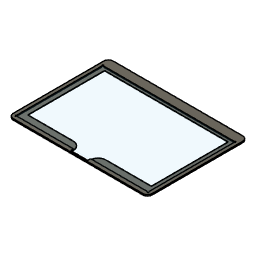
Pixsso_Assembly (Autodesk Fusion 360 archive; units mm, degrees)
design "PixssoFrame_ScreenBack"
Autodesk Fusion 360 part; units mm, degrees
sketch "Sketch1" plane through (0, 0, 0) normal (0, 0, 1) x (1, 0, 0)
  line L0 (90, 64.7) -> (-90, 64.7)
  line L1 (-90, 64.7) -> (-90, -64.7)
  line L2 (-90, -64.7) -> (90, -64.7)
  line L3 (90, -64.7) -> (90, 64.7)
  line L4 (90, 64.7) -> (-90, -64.7) construction
  line L5 (-90, 64.7) -> (90, -64.7) construction
  dimension "d1" = 129.4
  dimension "d2" = 180
  constraint horizontal L0
  constraint perpendicular L0 L1
  constraint parallel L0 L2
  constraint parallel L1 L3
  constraint coincident L4 origin
  constraint coincident L5 origin
  measures "d1" distance of L0.end L1.end
  measures "d2" distance of L0.start L0.end
extrude "Extrude1" add sketch "Sketch1" along normal blind 0.4
sketch "Sketch2" plane through (0, 0, 0.4) normal (0, 0, 1) x (-1, 0, 0)
  line L0 (-90, 64.7) -> (-90, -64.7)
  line L1 (-90, -64.7) -> (90, -64.7)
  line L2 (90, -64.7) -> (90, 64.7)
  line L3 (90, 64.7) -> (-90, 64.7)
  line L4 (90, -64.7) -> (-90, -64.7)
  line L5 (-90, -64.7) -> (-90, 64.7)
  line L6 (-90, 64.7) -> (90, 64.7)
  line L7 (90, 64.7) -> (90, -64.7)
  line L8 (85.65, -52.95) -> (-85.65, -52.95)
  line L9 (-85.65, -52.95) -> (-85.65, 59.55)
  line L10 (-85.65, 59.55) -> (85.65, 59.55)
  line L11 (85.65, 59.55) -> (85.65, -52.95)
  line L12 (0, -64.7) -> (0, -52.95) construction
  dimension "d5" = 112.5
  dimension "d6" = 171.3
  dimension "d7" = 5.15
  constraint horizontal L4
  constraint vertical L5
  constraint horizontal L6
  constraint vertical L7
  constraint coincident L0.start L3.end
  constraint coincident L1.end L2.start
  constraint horizontal L8
  constraint vertical L9
  constraint horizontal L10
  constraint vertical L11
  constraint midpoint L1 L12.start
  constraint midpoint L8 L12.end
  constraint vertical L12
  measures "d5" distance of L8.start L10.end
  measures "d6" distance of L8.start L8.end
  measures "d7" distance of L6 L10
extrude "Extrude2" add sketch "Sketch2" along normal blind 1.2
sketch "Sketch3" plane through (0, 0, 0.4) normal (0, 0, 1) x (-1, 0, 0)
  line L0 (-85.65, 59.55) -> (-85.65, -52.95)
  line L1 (-85.65, -52.95) -> (85.65, -52.95)
  line L2 (85.65, -52.95) -> (85.65, 59.55)
  line L3 (85.65, 59.55) -> (-85.65, 59.55)
sketch "Sketch4" plane through (0, 0, 0.4) normal (0, 0, 1) x (-1, 0, 0)
  line L0 (-80, -49.7) -> (80, -49.7)
  line L1 (80, -49.7) -> (80, 49.7)
  line L2 (80, 49.7) -> (-80, 49.7)
  line L3 (-80, 49.7) -> (-80, -49.7)
  line L4 (-80, -49.7) -> (80, 49.7) construction
  line L5 (80, -49.7) -> (-80, 49.7) construction
  point P0 (-90, -64.7)
  dimension "d10" = 15
  dimension "d11" = 10
  constraint horizontal L0
  constraint perpendicular L0 L1
  constraint parallel L0 L2
  constraint parallel L1 L3
  constraint coincident L4 origin
  constraint coincident L5 origin
  measures "d10" vertical distance of L0.start P0
  measures "d11" distance of L3 P0
extrude "Extrude3" cut sketch "Sketch4" against normal through all
sketch "Sketch5" plane through (0, 0, 1.6) normal (0, 0, 1) x (-1, 0, 0)
  line L0 (-85.65, 59.55) -> (85.65, 59.55)
  line L1 (85.65, 59.55) -> (85.65, -52.95)
  line L2 (85.65, -52.95) -> (-85.65, -52.95)
  line L3 (-85.65, -52.95) -> (-85.65, 59.55)
  line L4 (90, 64.7) -> (-90, 64.7)
  line L5 (-90, 64.7) -> (-90, -64.7)
  line L6 (-90, -64.7) -> (90, -64.7)
  line L7 (90, -64.7) -> (90, 64.7)
  line L8 (-11, 63.2) -> (11, 63.2)
  line L9 (11, 63.2) -> (11, 5)
  line L10 (11, 5) -> (-11, 5)
  line L11 (-11, 5) -> (-11, 63.2)
  line L12 (-11, 63.2) -> (11, 5) construction
  line L13 (11, 63.2) -> (-11, 5) construction
  line L14 (0, 5) -> (0, 0) construction
  point P0 (0, 34.1)
  dimension "d13" = 1.5
  dimension "d14" = 22
  dimension "d15" = 5
  constraint horizontal L8
  constraint perpendicular L8 L9
  constraint parallel L8 L10
  constraint parallel L9 L11
  constraint coincident L12 P0
  constraint coincident L13 P0
  constraint midpoint L10 L14.start
  constraint coincident L14.end origin
  constraint vertical L14
  measures "d13" distance of L4 L8
  measures "d14" distance of L8.start L8.end
  measures "d15" distance of L14.start L14.end
extrude "Extrude4" cut sketch "Sketch5" against normal through all contours L0 L8 L9 L11 | L0 L9 L10 L11
fillet "Fillet1" radius 10 2 edges at (-11, -49.7, 0.2) (11, -49.7, 0.2)
sketch "Sketch6" plane through (0, 0, 1.6) normal (0, 0, 1) x (-1, 0, 0)
  line L0 (90, 64.7) -> (-90, 64.7)
  line L1 (-90, 64.7) -> (-90, -64.7)
  line L2 (-90, -64.7) -> (90, -64.7)
  line L3 (90, -64.7) -> (90, 64.7)
  line L4 (-11, 59.7) -> (-11, 63.2)
  line L5 (-11, 63.2) -> (11, 63.2)
  line L6 (11, 63.2) -> (11, 59.7)
  line L7 (11.0011, 59.55) -> (85.65, 59.55)
  line L8 (85.65, 59.55) -> (85.65, -52.95)
  line L9 (85.65, -52.95) -> (-85.65, -52.95)
  line L10 (-85.65, -52.95) -> (-85.65, 59.55)
  line L11 (-85.65, 59.55) -> (-11.0011, 59.55)
  circle A0 centre (85.65, -52.95) radius 1
  circle A1 centre (85.65, 59.55) radius 1
  circle A2 centre (-85.65, 59.55) radius 1
  circle A3 centre (-85.65, -52.95) radius 1
  arc A4 (-11.0011, 59.55) -> (-11, 59.7) centre (-21, 59.7) ccw
  arc A5 (11, 59.7) -> (11.0011, 59.55) centre (21, 59.7) ccw
  dimension "d19" = 2
  constraint coincident L8.end L9.start
  constraint coincident L7.end L8.start
  constraint coincident L10.end L11.start
  constraint coincident L9.end L10.start
  constraint equal A0 A3
  constraint equal A2 A3
  constraint equal A1 A2
  measures "d19" diameter of A3
extrude "Extrude5" cut sketch "Sketch6" against normal up to surface (1.2 mm away) contours L10 L11 A2 | L9 L10 A3 | L7 L8 A1 | L8 L9 A0 picked at (-86.1315, 59.0916) picked at (-86.0843, -53.4534) picked at (86.2688, 59.7929) picked at (84.9871, -52.9997)
fillet "Fillet2" radius 6 4 edges at (90, -64.7, 0.8) (-90, -64.7, 0.8) (-90, 64.7, 0.8) (90, 64.7, 0.8)
equation "d7 = 4.9 mm + 0.25 mm"

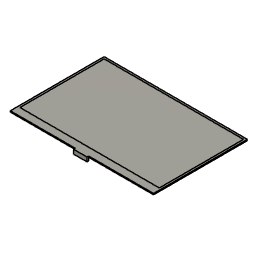
design "Waveshare_75in_eInkDisplay"
Autodesk Fusion 360 part; units mm, degrees
sketch "Sketch1" plane through (0, 0, 0) normal (0, 0, 1) x (1, 0, 0)
  line L0 (85, 55.65) -> (-85, 55.65)
  line L1 (-85, 55.65) -> (-85, -55.65)
  line L2 (-85, -55.65) -> (85, -55.65)
  line L3 (85, -55.65) -> (85, 55.65)
  line L4 (85, 55.65) -> (-85, -55.65) construction
  line L5 (-85, 55.65) -> (85, -55.65) construction
  dimension "d1" = 170
  dimension "d2" = 111.3
  constraint horizontal L0
  constraint perpendicular L0 L1
  constraint parallel L0 L2
  constraint parallel L1 L3
  constraint coincident L4 origin
  constraint coincident L5 origin
  measures "d1" distance of L0.start L0.end
  measures "d2" distance of L0.end L1.end
extrude "Extrude1" add sketch "Sketch1" along normal mid plane 1.3
sketch "Sketch2" plane through (0, 0, 0.65) normal (0, 0, 1) x (-1, 0, 0)
  line L0 (-85, 55.65) -> (-85, -55.65)
  line L1 (-85, -55.65) -> (85, -55.65)
  line L2 (85, -55.65) -> (85, 55.65)
  line L3 (85, 55.65) -> (-85, 55.65)
  line L4 (-82.7, -53.35) -> (82.7, -53.35)
  line L5 (82.7, -53.35) -> (82.7, 46.55)
  line L6 (82.7, 46.55) -> (-82.7, 46.55)
  line L7 (-82.7, 46.55) -> (-82.7, -53.35)
  line L8 (-82.7, -53.35) -> (82.7, 46.55) construction
  line L9 (82.7, -53.35) -> (-82.7, 46.55) construction
  line L10 (0, -3.4) -> (0, 0) construction
  point P0 (0, -3.4)
  dimension "d5" = 165.4
  dimension "d6" = 99.9
  dimension "d7" = 2.3
  constraint horizontal L4
  constraint perpendicular L4 L5
  constraint parallel L4 L6
  constraint parallel L5 L7
  constraint coincident L8 P0
  constraint coincident L9 P0
  constraint coincident P0 L10.start
  constraint coincident L10.end origin
  constraint vertical L10
  measures "d5" distance of L4.start L4.end
  measures "d6" distance of L4.end L5.end
  measures "d7" distance of L1 L4
extrude "Extrude2" cut sketch "Sketch2" against normal blind 0.001 contours L4 L5 L6 L7
sketch "Sketch3" plane through (0, 0, 0.65) normal (0, 0, 1) x (-1, 0, 0)
  line L0 (82.7, -53.35) -> (-82.7, -53.35)
  line L1 (-82.7, -53.35) -> (-82.7, 46.55)
  line L2 (-82.7, 46.55) -> (82.7, 46.55)
  line L3 (82.7, 46.55) -> (82.7, -53.35)
  line L4 (-85, 55.65) -> (-85, -55.65)
  line L5 (-85, -55.65) -> (85, -55.65)
  line L6 (85, -55.65) -> (85, 55.65)
  line L7 (85, 55.65) -> (-85, 55.65)
  line L8 (8, 55.65) -> (-8, 55.65)
  line L9 (-8, 55.65) -> (-8, 57.65)
  line L10 (-8, 57.65) -> (8, 57.65)
  line L11 (8, 57.65) -> (8, 55.65)
  line L12 (0, 55.65) -> (0, 0) construction
  dimension "d10" = 16
  dimension "d11" = 2
  constraint horizontal L8
  constraint vertical L9
  constraint horizontal L10
  constraint vertical L11
  constraint coincident L7 L8.start
  constraint midpoint L8 L12.start
  constraint coincident L12.end origin
  constraint vertical L12
  measures "d10" distance of L9.end L10.end
  measures "d11" distance of L8.end L9.end
extrude "Extrude3" add sketch "Sketch3" against normal blind 5 contours L7 L8 L9 L10 L11

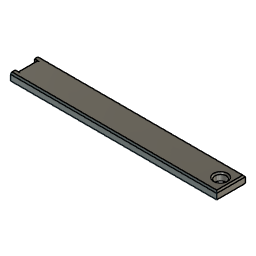
design "PixssoFrame_BatteryBracket"
Autodesk Fusion 360 part; units mm, degrees
sketch "Sketch1" plane through (0, 0, 0) normal (0, 0, 1) x (1, 0, 0)
  circle A0 centre (0, 0) radius 1.6
  line L0 (3, -4.1) -> (-55.8, -4.1)
  line L1 (-55.8, -4.1) -> (-55.8, 4.1)
  line L2 (-55.8, 4.1) -> (3, 4.1)
  line L3 (3, 4.1) -> (3, -4.1)
  line L4 (3, -4.1) -> (-55.8, 4.1) construction
  line L5 (-55.8, -4.1) -> (3, 4.1) construction
  point P0 (-26.4, 0)
  dimension "d1" = 55.8
  dimension "d2" = 3
  dimension "d3" = 3.2
  dimension "d4" = 8.2
  constraint coincident A0.centre origin
  constraint horizontal L0
  constraint perpendicular L0 L1
  constraint parallel L0 L2
  constraint parallel L1 L3
  constraint coincident L4 P0
  constraint coincident L5 P0
  constraint horizontal A0.centre P0
  measures "d1" distance of A0.centre L1
  measures "d2" distance of A0.centre L3
  measures "d3" diameter of A0
  measures "d4" distance of L0.start L2.end
extrude "Extrude1" add sketch "Sketch1" along normal blind 2
sketch "Sketch2" plane through (0, -4.1, 0) normal (0, -1, 0) x (1, 0, 0)
  line L0 (-55.8, 0) -> (3, 0)
  line L1 (3, 0) -> (3, 2)
  line L2 (3, 2) -> (-55.8, 2)
  line L3 (-55.8, 2) -> (-55.8, 0)
ref_plane "WorkPlane1" through (-26.4, 0, 1) normal (0, 1, 0) x (-1, 0, 0)
sketch "Sketch3" plane through (0, 0, 0) normal (0, 1, 0) x (1, 0, 0)
  line L0 (-55.8, 0) -> (-53.6, -1.2702)
  line L1 (-53.6, -1.2702) -> (-55.8, -2.5403)
  line L2 (-55.8, -2.5403) -> (-55.8, 0)
  line L3 (-55.8, 0) -> (3, 0)
  dimension "d7" = 30
  dimension "d8" = 30
  dimension "d9" = 2.2
  constraint vertical L2
  constraint coincident L0.start L2.end
  measures "d7" angle of L0 L3
  measures "d8" angle of L1 L3
  measures "d9" horizontal distance of L0.end L0.start
extrude "Extrude2" cut sketch "Sketch3" along normal mid plane 5.5
chamfer "Chamfer1" distance 0.4 distance2 0.4 4 edges at (-1.4917, 0.5786, 2) (-26.4, 4.1, 2) (3, 0, 2) (-26.4, -4.1, 2) measured on face at (-37.1094, 0, 2) measured on face at (-37.1094, 0, 2) measured on face at (-37.1094, 0, 2) measured on face at (-37.1094, 0, 2)

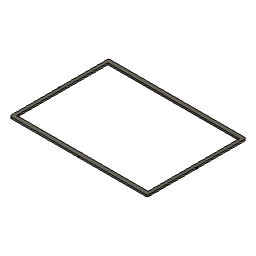
design "PixssoFrame_GlassSpacer"
Autodesk Fusion 360 part; units mm, degrees
sketch "Sketch1" plane through (0, 0, 0) normal (0, 0, 1) x (1, 0, 0)
  line L0 (89, 64) -> (-89, 64)
  line L1 (-89, 64) -> (-89, -64)
  line L2 (-89, -64) -> (89, -64)
  line L3 (89, -64) -> (89, 64)
  line L4 (89, 64) -> (-89, -64) construction
  line L5 (-89, 64) -> (89, -64) construction
  line L6 (84.9, 58.9) -> (-84.9, 58.9)
  line L7 (-84.9, 58.9) -> (-84.9, -58.9)
  line L8 (-84.9, -58.9) -> (84.9, -58.9)
  line L9 (84.9, -58.9) -> (84.9, 58.9)
  line L10 (84.9, 58.9) -> (-84.9, -58.9) construction
  line L11 (-84.9, 58.9) -> (84.9, -58.9) construction
  dimension "d1" = 128
  dimension "d2" = 178
  dimension "d3" = 4.1
  dimension "d4" = 5.1
  dimension "d12" = 117.8
  constraint horizontal L0
  constraint perpendicular L0 L1
  constraint parallel L0 L2
  constraint parallel L1 L3
  constraint coincident L4 origin
  constraint coincident L5 origin
  constraint horizontal L6
  constraint perpendicular L6 L7
  constraint parallel L6 L8
  constraint parallel L7 L9
  constraint coincident L10 origin
  constraint coincident L11 origin
  measures "d1" distance of L0.end L1.end
  measures "d2" distance of L0.start L0.end
  measures "d3" distance of L3 L9
  measures "d4" distance of L0 L6
  measures "d12" distance of L6 L8
extrude "Extrude1" add sketch "Sketch1" along normal blind 2
fillet "Fillet1" radius 2 4 edges at (89, -64, 1) (-89, -64, 1) (89, 64, 1) (-89, 64, 1)
sketch "Sketch2" plane through (0, 0, 2) normal (0, 0, 1) x (-1, 0, 0)
  line L0 (-84.9, -58.9) -> (-84.9, 58.9)
  line L1 (-84.9, 58.9) -> (84.9, 58.9)
  line L2 (84.9, 58.9) -> (84.9, -58.9)
  line L3 (84.9, -58.9) -> (-84.9, -58.9)
  arc A0 (87, -64) -> (89, -62) centre (87, -62) ccw
  line L4 (89, -62) -> (89, 62)
  arc A1 (89, 62) -> (87, 64) centre (87, 62) ccw
  line L5 (87, 64) -> (-87, 64)
  arc A2 (-87, 64) -> (-89, 62) centre (-87, 62) ccw
  line L6 (-89, 62) -> (-89, -62)
  arc A3 (-89, -62) -> (-87, -64) centre (-87, -62) ccw
  line L7 (-87, -64) -> (87, -64)
  line L8 (0, -64) -> (0, -64.7) construction
  line L9 (0, -64.7) -> (0.7, -64)
  line L10 (0.7, -64) -> (0, -64)
  line L11 (89, 0) -> (89, -0.7)
  line L12 (89, -0.7) -> (89.7, 0)
  line L13 (89.7, 0) -> (89, 0.7)
  line L14 (89, 0.7) -> (89, 0)
  line L15 (0, -64.7) -> (-0.7, -64)
  line L16 (0, -64) -> (-0.7, -64)
  line L17 (84.9, 0) -> (0, 0) construction
  line L18 (0, 64.7) -> (0.7, 64)
  line L19 (0, 64.7) -> (-0.7, 64)
  line L20 (0, 64) -> (-0.7, 64)
  line L21 (0.7, 64) -> (0, 64)
  line L22 (-89, -0.7) -> (-89.7, 0)
  line L23 (-89.7, 0) -> (-89, 0.7)
  line L24 (-89, 0.7) -> (-89, 0)
  line L25 (-89, 0) -> (-89, -0.7)
  dimension "d9" = 129.4
  constraint midpoint L7 L8.start
  constraint perpendicular L7 L8
  constraint coincident L7 L9.end
  constraint midpoint L4 L11.start
  constraint coincident L4 L11.end
  constraint perpendicular L3 L11
  constraint parallel L9 L12
  constraint coincident L4 L13.end
  constraint coincident L7 L15.end
  constraint equal L10 L16
  constraint equal L11 L16
  constraint equal L11 L14
  constraint equal L12 L15
  constraint equal L12 L13
  constraint midpoint L2 L17.start
  constraint coincident L17.end origin
  constraint symmetric L8.start L17 L20.start
  constraint symmetric L8.end L17 L18.start
  constraint symmetric L9.end L17 L18.end
  constraint symmetric L15.end L17 L19.end
  constraint symmetric L8 L11.start L24.end
  constraint symmetric L8 L11.end L22.start
  constraint symmetric L8 L12.end L22.end
  constraint symmetric L8 L13.end L23.end
  measures "d9" distance of L8.end L18.start
extrude "Extrude2" add sketch "Sketch2" against normal up to surface (2 mm away) contours L7 L9 L10 L15 L16 | L4 L11 L12 L13 L14 | L6 L22 L23 L24 L25 | L5 L18 L19 L20 L21
equation "d1 = 126.5 mm + 1.5 mm"
equation "d2 = 176 mm + 2 mm"

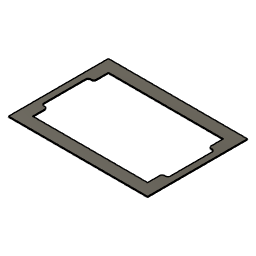
design "PixssoFrame_PaperFrame"
Autodesk Fusion 360 part; units mm, degrees
sketch "Sketch1" plane through (0, 0, 0) normal (0, 0, 1) x (1, 0, 0)
  line L0 (89.5, 64.25) -> (-89.5, 64.25)
  line L1 (-89.5, 64.25) -> (-89.5, -64.25)
  line L2 (-89.5, -64.25) -> (89.5, -64.25)
  line L3 (89.5, -64.25) -> (89.5, 64.25)
  line L4 (89.5, 64.25) -> (-89.5, -64.25) construction
  line L5 (-89.5, 64.25) -> (89.5, -64.25) construction
  dimension "d1" = 179
  dimension "d2" = 128.5
  constraint horizontal L0
  constraint perpendicular L0 L1
  constraint parallel L0 L2
  constraint parallel L1 L3
  constraint coincident L4 origin
  constraint coincident L5 origin
  measures "d1" distance of L1.end L2.end
  measures "d2" distance of L0.start L2.end
extrude "Extrude1" add sketch "Sketch1" along normal mid plane 1
sketch "Sketch2" plane through (0, 0, 0.5) normal (0, 0, 1) x (-1, 0, 0)
  line L0 (-89.5, 64.25) -> (-89.5, -64.25)
  line L1 (-89.5, -64.25) -> (89.5, -64.25)
  line L2 (89.5, -64.25) -> (89.5, 64.25)
  line L3 (89.5, 64.25) -> (-89.5, 64.25)
  line L4 (0, 0) -> (81.4, 0) construction
  line L5 (81.4, 0) -> (81.4, -30)
  line L6 (81.4, -30) -> (74, -30)
  line L7 (74, -30) -> (74, -48.75)
  line L8 (74, -48.75) -> (0, -48.75)
  line L9 (0, -48.75) -> (0, 0) construction
  line L10 (81.4, 30) -> (74, 30)
  line L11 (74, 30) -> (74, 48.75)
  line L12 (81.4, 0) -> (81.4, 30)
  line L13 (74, 48.75) -> (0, 48.75)
  line L14 (-81.4, 0) -> (-81.4, 30)
  line L15 (-81.4, 0) -> (-81.4, -30)
  line L16 (-74, 30) -> (-74, 48.75)
  line L17 (-81.4, -30) -> (-74, -30)
  line L18 (-81.4, 30) -> (-74, 30)
  line L19 (-74, -30) -> (-74, -48.75)
  line L20 (-74, -48.75) -> (0, -48.75)
  line L21 (-74, 48.75) -> (0, 48.75)
  line L22 (74, -64.25) -> (74, -48.75) construction
  line L23 (89.5, -48.75) -> (74, -48.75) construction
  point P0 (89.5, 64.25)
  point P1 (-89.5, -64.25)
  dimension "d5" = 97.5
  dimension "d7" = 162.8
  dimension "d8" = 60
  constraint coincident L4.start L9.end
  constraint horizontal L4
  constraint perpendicular L4 L5
  constraint perpendicular L5 L6
  constraint perpendicular L6 L7
  constraint perpendicular L7 L8
  constraint perpendicular L4 L9
  constraint symmetric L1.end L4 P0
  constraint symmetric L5.start L4 L12.start
  constraint symmetric L4 L5.end L10.start
  constraint symmetric L4 L6.end L10.end
  constraint symmetric L4 L7.end L11.end
  constraint symmetric L4 L8.end L13.end
  constraint symmetric L1.end L9 P1
  constraint symmetric L4.end L9 L14.start
  constraint symmetric L5.end L9 L15.end
  constraint symmetric L6.end L9 L17.end
  constraint symmetric L7.end L9 L19.end
  constraint symmetric L8.end L9 L20.end
  constraint symmetric L9 L10.start L14.end
  constraint symmetric L9 L11.end L16.end
  constraint symmetric L9 L10.end L16.start
  constraint symmetric L9 L4.end L14.start
  constraint symmetric L9 L13.end L21.end
  constraint coincident L1 L22.start
  constraint perpendicular L8 L22
  constraint coincident L2 L23.start
  constraint perpendicular L22 L23
  constraint equal L22 L23
  measures "d5" distance of L20 L21
  measures "d7" distance of L5 L15
  measures "d8" distance of L5.end L10.start
extrude "Extrude2" cut sketch "Sketch2" against normal through all contours L5 L6 L7 L8 L10 L11 L12 L13 L14 L15 L16 L17 L18 L19 L20 L21
fillet "Fillet1" radius 3 8 edges at (-74, 30, 0) (-81.4, 30, 0) (-81.4, -30, 0) (-74, -30, 0) (74, -30, 0) (81.4, -30, 0) (74, 30, 0) (81.4, 30, 0)
equation "d7 = 163.2 mm - 0.4 mm"

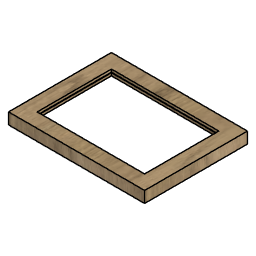
design "PixssoFrame_WoodFrame"
Autodesk Fusion 360 part; units mm, degrees
sketch "Sketch1" plane through (0, 0, 0) normal (0, 0, 1) x (1, 0, 0)
  line L0 (104.5, 79) -> (-104.5, 79)
  line L1 (-104.5, 79) -> (-104.5, -79)
  line L2 (-104.5, -79) -> (104.5, -79)
  line L3 (104.5, -79) -> (104.5, 79)
  line L4 (104.5, 79) -> (-104.5, -79) construction
  line L5 (-104.5, 79) -> (104.5, -79) construction
  line L6 (82.5, 57) -> (-82.5, 57)
  line L7 (-82.5, 57) -> (-82.5, -57)
  line L8 (-82.5, -57) -> (82.5, -57)
  line L9 (82.5, -57) -> (82.5, 57)
  line L10 (82.5, 57) -> (-82.5, -57) construction
  line L11 (-82.5, 57) -> (82.5, -57) construction
  dimension "d1" = 209
  dimension "d2" = 158
  dimension "d3" = 165
  dimension "d4" = 114
  constraint horizontal L0
  constraint perpendicular L0 L1
  constraint parallel L0 L2
  constraint parallel L1 L3
  constraint coincident L4 origin
  constraint coincident L5 origin
  constraint horizontal L6
  constraint perpendicular L6 L7
  constraint parallel L6 L8
  constraint parallel L7 L9
  constraint coincident L10 origin
  constraint coincident L11 origin
  measures "d1" distance of L0.start L0.end
  measures "d2" distance of L0.start L2.end
  measures "d3" distance of L7.end L8.end
  measures "d4" distance of L6.end L7.end
  measures "d13" distance of L7.end
extrude "Extrude1" add sketch "Sketch1" along normal mid plane 17.3
sketch "Sketch2" plane through (0, 0, -8.65) normal (0, 0, -1) x (1, 0, 0)
  line L0 (82.5, 57) -> (82.5, -57)
  line L1 (82.5, -57) -> (-82.5, -57)
  line L2 (-82.5, -57) -> (-82.5, 57)
  line L3 (-82.5, 57) -> (82.5, 57)
  line L4 (104.5, -79) -> (104.5, 79)
  line L5 (104.5, 79) -> (-104.5, 79)
  line L6 (-104.5, 79) -> (-104.5, -79)
  line L7 (-104.5, -79) -> (104.5, -79)
  line L8 (-90.75, -65.25) -> (90.75, -65.25)
  line L9 (90.75, -65.25) -> (90.75, 65.25)
  line L10 (90.75, 65.25) -> (-90.75, 65.25)
  line L11 (-90.75, 65.25) -> (-90.75, -65.25)
  line L12 (-90.75, -65.25) -> (90.75, 65.25) construction
  line L13 (90.75, -65.25) -> (-90.75, 65.25) construction
  dimension "d7" = 181.5
  dimension "d8" = 130.5
  constraint horizontal L8
  constraint perpendicular L8 L9
  constraint parallel L8 L10
  constraint parallel L9 L11
  constraint coincident L12 origin
  constraint coincident L13 origin
  measures "d7" distance of L8.start L8.end
  measures "d8" distance of L8.start L10.end
extrude "Extrude2" cut sketch "Sketch2" against normal blind 13.1 contours L0 L1 L2 L3 | L8 L9 L10 L11
ref_plane "WorkPlane1" through (0, 0, -1.95) normal (0, 0, -1) x (-1, 0, 0)
sketch "Sketch3" plane through (0, 0, -1.95) normal (0, 0, -1) x (-1, 0, 0)
  line L0 (93.75, 68.25) -> (-93.75, 68.25)
  line L1 (-93.75, 68.25) -> (-93.75, -68.25)
  line L2 (-93.75, -68.25) -> (93.75, -68.25)
  line L3 (93.75, -68.25) -> (93.75, 68.25)
  line L4 (93.75, 68.25) -> (-93.75, -68.25) construction
  line L5 (-93.75, 68.25) -> (93.75, -68.25) construction
  dimension "d12" = 187.5
  dimension "d13" = 136.5
  constraint horizontal L0
  constraint perpendicular L0 L1
  constraint parallel L0 L2
  constraint parallel L1 L3
  constraint coincident L4 origin
  constraint coincident L5 origin
  measures "d12" distance of L1.end L2.end
  measures "d13" distance of L0.start L2.end
extrude "Extrude3" cut sketch "Sketch3" along normal blind 2.5
